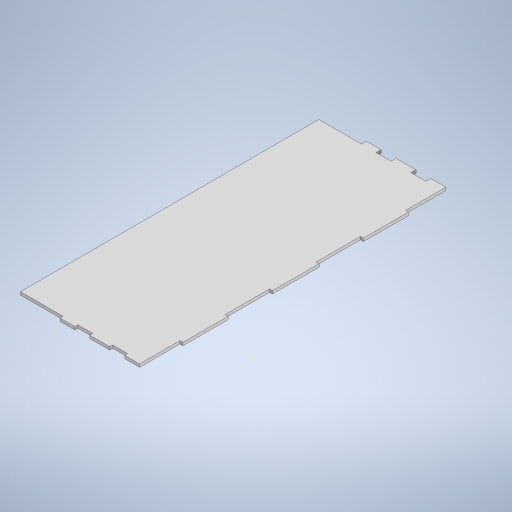
# Autodesk Inventor part: mieng_ben_3mm
Saved by Autodesk Inventor 2023 (Build 270158000, 158)
## iProperties
Created: 2022-11-20
Part Number: mieng_ben_3mm
Material: Generic
Document SubType Name: Modeling
Designer: ADMIN
Density: 1 g/cm^3
Appearance: Default
Author: ADMIN
Autodesk Inventor part; units mm, degrees
ref_plane "YZ Plane" through (0, 0, 0) normal (1, 0, 0) x (0, 1, 0)
ref_plane "XZ Plane" through (0, 0, 0) normal (0, 1, 0) x (-1, 0, 0)
ref_plane "XY Plane" through (0, 0, 0) normal (0, 0, 1) x (1, 0, 0)
sketch "Sketch1" plane through (0, 0, 0) normal (0, 1, 0) x (-1, 0, 0)
  point P0 (0, 0)
sketch "Sketch3" plane through (0, 0, 0) normal (0, 1, 0) x (-1, 0, 0)
  line L0 (113.8824, -237.8336) -> (98.8824, -237.8336)
  line L1 (128.8824, -242.8336) -> (113.8824, -242.8336)
  line L2 (128.8824, -242.8336) -> (128.8824, -237.8336)
  line L3 (98.8824, -237.8336) -> (98.8824, -242.8336)
  line L4 (113.8824, -242.8336) -> (113.8824, -237.8336)
  line L5 (48.8824, -156.8908) -> (45.8824, -156.8908)
  line L6 (48.8824, -156.8908) -> (48.8824, -112.2516)
  line L7 (48.8824, -112.2516) -> (45.8824, -112.2516)
  line L8 (45.8824, -112.2516) -> (45.8824, -65.4156)
  line L9 (48.8824, -65.4156) -> (45.8824, -65.4156)
  line L10 (48.8824, -156.8908) -> (48.8824, -112.2516)
  line L11 (98.8824, -242.8336) -> (78.8824, -242.8336)
  line L12 (63.8824, -237.8336) -> (75.0605, -237.8336)
  line L13 (48.8824, -237.8336) -> (48.8824, -202.2369)
  line L14 (48.8824, -202.2369) -> (45.8824, -202.2369)
  line L15 (45.8824, -202.2369) -> (45.8824, -156.8908)
  line L16 (48.8824, -20.7764) -> (45.8824, -20.7764)
  line L17 (45.8824, -20.7764) -> (45.8824, 24.5697)
  line L18 (48.8824, -65.4156) -> (48.8824, -20.7764)
  line L19 (48.8824, -65.4156) -> (48.8824, -20.7764)
  line L20 (48.8824, 24.5697) -> (45.8824, 24.5697)
  line L21 (113.8824, 65.1664) -> (113.8824, 62.1664)
  line L22 (48.8824, 24.5697) -> (48.8824, 62.1664)
  line L23 (48.8824, 24.5697) -> (48.8824, 65.1664)
  line L24 (48.8824, 65.1664) -> (63.8824, 65.1664)
  line L25 (63.8824, 62.1664) -> (78.8824, 62.1664)
  line L26 (63.8824, 65.1664) -> (63.8824, 62.1664)
  line L27 (78.8824, 62.1664) -> (78.8824, 65.1664)
  line L28 (78.8824, 65.1664) -> (98.8824, 65.1664)
  line L29 (98.8824, 62.1664) -> (98.8824, 65.1664)
  line L30 (98.8824, 62.1664) -> (113.8824, 62.1664)
  line L31 (128.8824, 62.1664) -> (128.8824, 65.1664)
  line L32 (113.8824, 65.1664) -> (128.8824, 65.1664)
  line L33 (63.8824, -237.8336) -> (78.8824, -237.8336)
  line L34 (48.8824, -242.8336) -> (48.8824, -237.8336)
  line L35 (48.8824, -242.8336) -> (63.8824, -242.8336)
  line L36 (63.8824, -242.8336) -> (63.8824, -237.8336)
  line L37 (78.8824, -237.8336) -> (78.8824, -242.8336)
  line L38 (78.8824, -237.8336) -> (63.8824, -237.8336)
  line L39 (171.6524, -88.8336) -> (171.6524, -237.8336)
  line L40 (171.6524, -237.8336) -> (128.8824, -237.8336)
  line L41 (171.6524, -88.8336) -> (171.6524, 62.1664)
  line L42 (171.6524, 62.1664) -> (128.8824, 62.1664)
  point P0 (0, 0)
  point P1 (0, 0)
  point P2 (106.3824, -237.8336)
  point P3 (47.3824, -202.2369)
  point P4 (0, 0)
  point P5 (106.3824, 62.1664)
  point P6 (121.3824, 65.1664)
  dimension "d54" = 80
  dimension "d55" = 15
  dimension "d56" = 15
  dimension "d57" = 300
  dimension "d58" = 3
  dimension "d59" = 5
  dimension "d60" = 44.6392
  dimension "d61" = 37.5967
  dimension "d62" = 44.6392
  dimension "d63" = 40.5967
  dimension "d64" = 45.3461
  dimension "d66" = 45.3461
  dimension "d67" = 20
  dimension "d68" = 15
  dimension "d69" = 15
  dimension "d70" = 15
  dimension "d71" = 15
  dimension "d72" = 15
  dimension "d73" = 15
  dimension "d74" = 20
  dimension "d75" = 308
  constraints: 86 end point, 16 perpendicular, 5 horizontal, 4 midpoint, 4 parallel, 2 point on line, 2 vertical
  measures "d54" distance of L2.end L13.start
  measures "d55" distance of L35.start L36.start
  measures "d56" distance of L33.start L37.start
  measures "d57" distance of point (106.382, -237.834) point (106.382, 62.166)
  measures "d58" vertical distance of L21.end point (121.382, 65.166)
  measures "d59" distance between parallel lines of L0 L1
  measures "d60" distance of L18.start L16.start
  measures "d61" distance of L23.start L22.end
  measures "d62" distance of L6.start L7.start
  measures "d63" distance from line of L35 point (47.382, -202.237)
  measures "d64" distance of L15.start L5.end
  measures "d66" distance of L16.end L20.end
  measures "d67" distance of L27.end L29.end
  measures "d68" distance of L29.start L21.end
  measures "d69" distance of L21.start L31.end
  measures "d70" distance of L24.start L24.end
  measures "d71" distance of L26.end L25.end
  measures "d72" distance of L1.start L1.end
  measures "d73" distance of L4.end L0.end
  measures "d74" distance of L3.end L11.end
  measures "d75" distance between parallel lines of L1 L32
extrude "Extrusion2" add sketch "Sketch3" along normal blind 3
body "Solid2"
